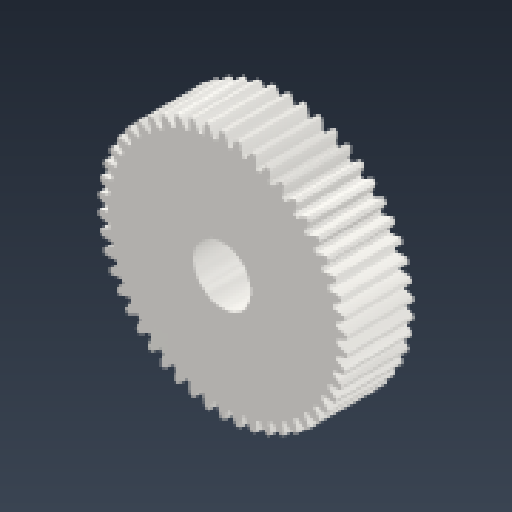
# Autodesk Inventor part: Цилиндрическое зубчатое зацепление1
Saved by Autodesk Inventor 2025 (Build 290162000, 162)
## iProperties
Created: 2025-09-21
Part Number: Цилиндрическое зубчатое зацепление1
Material: Steel
Document SubType Name: Modeling
Designer: GameHD
Categories: <?xml version="1.0" encoding="UTF-16"?> <MemberInstance><Categories><FamilyTemplate><FamilyTemplateParameter ValueType="xs:double" Id="1" ObjectReferenceKey="da_z" ObjectType="kUserParameterObject"/><FamilyTemplateParameter ValueType="xs:double" Id="2" ObjectReferenceKey="da_b" ObjectType="kUserParameterObject"/><FamilyTemplateParameter ValueType="xs:double" Id="3" ObjectReferenceKey="da_beta" ObjectType="kUserParameterObject"/><FamilyTemplateParameter ValueType="xs:double" Id="4" ObjectReferenceKey="da_da" ObjectType="kUserParameterObject"/><FamilyTemplateParameter ValueType="xs:double" Id="5" ObjectReferenceKey="da_aw" ObjectType="kUserParameterObject"/><FamilyTemplateParameter ValueType="xs:string" Id="6" ObjectReferenceKey="EAIAABAAAACIAQAAAAAAAIAAAAAAAAAA" ObjectType="83910656" SubObjectId="SurfaceGeometry"/></FamilyTemplate><ParamToTemplateMap><ParamToTemplate CategoryParameter="//CategoryParameter[@InternalName='046C89C9-8512-4d59-83FE-43B91F4F132A']" TemplateParameter="1"/><ParamToTemplate CategoryParameter="//CategoryParameter[@InternalName='2552DF32-E462-4b46-AEBF-C6C7768E72AC']" TemplateParameter="2"/><ParamToTemplate CategoryParameter="//CategoryParameter[@InternalName='C9EE641D-15FC-4fae-A226-E94C4372FDD7']" TemplateParameter="3"/><ParamToTemplate><ParamToTemplate CategoryParameter="//CategoryParameter[@InternalName='00B6519A-459B-49c7-AD84-2E56D39A5744']" ConstantValue="0.000000"/></ParamToTemplate><ParamToTemplate><ParamToTemplate CategoryParameter="//CategoryParameter[@InternalName='04B31F0E-C7A6-4894-AA32-9629BEFACF47']" ConstantValue="1.000000"/></ParamToTemplate><ParamToTemplate><ParamToTemplate CategoryParameter="//CategoryParameter[@InternalName='43CBEC2E-7847-49e7-A936-2F7889FCB2D9']" ConstantValue="0.250000"/></ParamToTemplate><ParamToTemplate><ParamToTemplate CategoryParameter="//CategoryParameter[@InternalName='B1EFC894-105D-4ebd-86BF-FA20ED196853']" ConstantValue="0.350000"/></ParamToTemplate><ParamToTemplate><ParamToTemplate CategoryParameter="//CategoryParameter[@InternalName='51175063-3D10-4879-93E8-6246FE8B403D']" ConstantValue="2060000000.000000"/></ParamToTemplate><ParamToTemplate><ParamToTemplate CategoryParameter="//CategoryParameter[@InternalName='A3A52E27-4454-46a9-B0BD-C932399B70AF']" ConstantValue="0.300000"/></ParamToTemplate><ParamToTemplate><ParamToTemplate CategoryParameter="//CategoryParameter[@InternalName='91B76062-C214-41d9-B1B9-14D2AB99603D']" ConstantValue="0.050000"/></ParamToTemplate><ParamToTemplate><ParamToTemplate CategoryParameter="//CategoryParameter[@InternalName='374E806E-8B8A-4dda-A9AA-1039D6500AD2']" ConstantValue="20.000000"/></ParamToTemplate><ParamToTemplate><ParamToTemplate CategoryParameter="//CategoryParameter[@InternalName='2D373A89-B862-43d6-8D0B-0CBF12AB9F6C']" ConstantValue="0.349066"/></ParamToTemplate><ParamToTemplate CategoryParameter="//CategoryParameter[@InternalName='37777632-D6A2-4fac-9D53-DB8ACD95C989']" TemplateParameter="4"/><ParamToTemplate CategoryParameter="//CategoryParameter[@InternalName='FD1017F1-B727-4f7e-9707-0F86F1FF9423']" TemplateParameter="5"/><ParamToTemplate><ParamToTemplate CategoryParameter="//CategoryParameter[@InternalName='9E1B4470-B2D3-4ff1-B813-535BB4CDF51A']" ConstantValue="3520000.000000"/></ParamToTemplate><ParamToTemplate><ParamToTemplate CategoryParameter="//CategoryParameter[@InternalName='F8452263-BFF6-458c-9FB1-07C4B99E95CD']" ConstantValue="11400000.000000"/></ParamToTemplate><ParamToTemplate><ParamToTemplate CategoryParameter="//CategoryParameter[@InternalName='3E3BB259-FD49-497f-8171-6EBC954A3479']" ConstantValue="2.000000"/></ParamToTemplate><ParamToTemplate CategoryParameter="//CategoryParameter[@InternalName='27C3BAF2-7550-4e4b-AE2C-0DB134B7D9B7']" TemplateParameter="6"/></ParamToTemplateMap><Category DisplayName="Gear" InternalName="DC85795E-93AB-48d5-8EEE-5A27447B64BD" Mnemonic="Gear"><CategoryParameter DisplayName="z" InternalName="046C89C9-8512-4d59-83FE-43B91F4F132A" Mnemonic="z"/><CategoryParameter DisplayName="b" InternalName="2552DF32-E462-4b46-AEBF-C6C7768E72AC" Mnemonic="b"/><CategoryParameter DisplayName="||b|" InternalName="C9EE641D-15FC-4fae-A226-E94C4372FDD7" Mnemonic="beta"/><CategoryParameter DisplayName="x" InternalName="00B6519A-459B-49c7-AD84-2E56D39A5744" Mnemonic="x"/><CategoryParameter DisplayName="a*" InternalName="04B31F0E-C7A6-4894-AA32-9629BEFACF47" Mnemonic="a"/><CategoryParameter DisplayName="c*" InternalName="43CBEC2E-7847-49e7-A936-2F7889FCB2D9" Mnemonic="c"/><CategoryParameter DisplayName="r|.f|*" InternalName="B1EFC894-105D-4ebd-86BF-FA20ED196853" Mnemonic="rf"/><CategoryParameter DisplayName="E" InternalName="51175063-3D10-4879-93E8-6246FE8B403D" Mnemonic="E"/><CategoryParameter DisplayName="||m|" InternalName="A3A52E27-4454-46a9-B0BD-C932399B70AF" Mnemonic="mi"/><Category DisplayName="SpurGear" InternalName="26C5A22E-A91E-4dfd-A3B3-23CCAFAE1764" Mnemonic="SpurGear"><CategoryParameter DisplayName="m" InternalName="91B76062-C214-41d9-B1B9-14D2AB99603D" Mnemonic="m"/><CategoryParameter DisplayName="P" InternalName="374E806E-8B8A-4dda-A9AA-1039D6500AD2" Mnemonic="PP"/><CategoryParameter DisplayName="||a|" InternalName="2D373A89-B862-43d6-8D0B-0CBF12AB9F6C" Mnemonic="alpha"/><CategoryParameter DisplayName="d|.a|" InternalName="37777632-D6A2-4fac-9D53-DB8ACD95C989" Mnemonic="da"/><CategoryParameter DisplayName="a|.w|" InternalName="FD1017F1-B727-4f7e-9707-0F86F1FF9423" Mnemonic="aw"/><CategoryParameter DisplayName="||s||.Flim|" InternalName="9E1B4470-B2D3-4ff1-B813-535BB4CDF51A" Mnemonic="sFlim"/><CategoryParameter DisplayName="||s||.Hlim|" InternalName="F8452263-BFF6-458c-9FB1-07C4B99E95CD" Mnemonic="sHlim"/><CategoryParameter DisplayName="тип" InternalName="3E3BB259-FD49-497f-8171-6EBC954A3479" Mnemonic="type"/><CategoryParameter DisplayName="PitchDiameter" InternalName="27C3BAF2-7550-4e4b-AE2C-0DB134B7D9B7" Mnemonic="IDS_PITCHDIAM"/></Category></Category></Categories></MemberInstance>
Density: 1 g/cm^3
Appearance: Steel
CustomPartVersion: 1
Author: GameHD
Autodesk Inventor part; units mm, degrees
sketch "Sketch1" plane through (0, 0, 0) normal (0, 0, 1) x (1, 0, 0)
  circle A0 centre (0, 0) radius 13
  dimension "d0" = 26
  constraints: 1 centre point
  measures "d0" diameter of A0
extrude "Extrusion1" add sketch "Sketch1" along normal blind 6.5
ref_plane "Work Plane2" through (0, 0, 3.25) normal (0, 0, 1) x (1, 0, 0)
sketch "Sketch2" plane through (0, 0, 0) normal (0, 0, -1) x (-1, 0, 0)
  circle A0 centre (0, 0) radius 13 projected
  circle A1 centre (0, 0) radius 12.5
  dimension "d3" = 25
  constraints: 1 centre point, 1 coincident
  measures "d3" diameter of A1
surface extrude "Средний диаметр" sketch "Sketch2" against normal through all shown no curves A1
ref_plane "Work Plane8" through (0, 0, 0) normal (0.9980267, 0.0627905, 0) x (0, 0, 1)
ref_plane "Work Plane9" through (0, 0, 0) normal (1, 0, 0) x (0, 1, 0)
spur gear teeth "Цилиндрическое зубчатое зацепление" teeth 50 pitch diameter 25 tip diameter 26 root diameter 23.75 face width 6.5 start plane through (0, 0, 0) normal (0, 0, -1) x (-1, 0, 0)
sketch "Эскиз3" plane through (0, 0, 6.5) normal (0, 0, 1) x (1, 0, 0)
  circle A0 centre (0, 0) radius 3
  dimension "d49" = 6
  constraints: 1 centre point, 1 coincident
  measures "d49" diameter of A0
extrude "Выдавливание2" cut sketch "Эскиз3" against normal blind 10
sketch "Эскиз4" plane through (0, 0, 6.5) normal (0, 0, 1) x (1, 0, 0)
  circle A0 centre (0, 0) radius 4.5
  circle A1 centre (0, 0) radius 3 projected
  dimension "d52" = 9
  constraints: 1 centre point, 1 coincident
  measures "d52" diameter of A0
extrude "Выдавливание3" add sketch "Эскиз4" along normal blind 1
sketch "Эскиз5" plane through (0, 0, 0) normal (0, 0, -1) x (-1, 0, 0)
  circle A0 centre (0, 0) radius 4.5 projected
  circle A1 centre (0, 0) radius 3 projected
  arc A2 (2.0417, 11.6982) -> (1.8317, 12.8703) centre (-3.9363, 11.2323) ccw projected
  arc A3 (1.8317, 12.8703) -> (1.4265, 12.9215) centre (0, 0) ccw projected
  arc A4 (1.4265, 12.9215) -> (0.9317, 11.8384) centre (6.606, 9.9005) ccw projected
  arc A5 (0.9317, 11.8384) -> (0.5594, 11.8618) centre (0, 0) ccw projected
  arc A6 (0.5594, 11.8618) -> (0.2042, 12.9984) centre (-5.313, 10.6504) ccw projected
  arc A7 (0.2042, 12.9984) -> (-0.2042, 12.9984) centre (0, 0) ccw projected
  arc A8 (-0.2042, 12.9984) -> (-0.5594, 11.8618) centre (5.313, 10.6504) ccw projected
  arc A9 (-0.5594, 11.8618) -> (-0.9317, 11.8384) centre (0, 0) ccw projected
  arc A10 (-0.9317, 11.8384) -> (-1.4265, 12.9215) centre (-6.606, 9.9005) ccw projected
  arc A11 (-1.4265, 12.9215) -> (-1.8317, 12.8703) centre (0, 0) ccw projected
  arc A12 (-1.8317, 12.8703) -> (-2.0417, 11.6982) centre (3.9363, 11.2323) ccw projected
  arc A13 (-2.0417, 11.6982) -> (-2.4081, 11.6283) centre (0, 0) ccw projected
  arc A14 (-2.4081, 11.6283) -> (-3.0348, 12.6408) centre (-7.7948, 8.9945) ccw projected
  arc A15 (-3.0348, 12.6408) -> (-3.4303, 12.5392) centre (0, 0) ccw projected
  arc A16 (-3.4303, 12.5392) -> (-3.4917, 11.35) centre (2.4975, 11.6371) ccw projected
  arc A17 (-3.4917, 11.35) -> (-3.8465, 11.2348) centre (0, 0) ccw projected
  arc A18 (-3.8465, 11.2348) -> (-4.5952, 12.1608) centre (-8.8606, 7.9466) ccw projected
  arc A19 (-4.5952, 12.1608) -> (-4.9749, 12.0104) centre (0, 0) ccw projected
  arc A20 (-4.9749, 12.0104) -> (-4.8867, 10.8229) centre (1.0193, 11.8584) ccw projected
  arc A21 (-4.8867, 10.8229) -> (-5.2243, 10.6641) centre (0, 0) ccw projected
  arc A22 (-5.2243, 10.6641) -> (-6.0831, 11.489) centre (-9.7867, 6.7734) ccw projected
  arc A23 (-6.0831, 11.489) -> (-6.441, 11.2922) centre (0, 0) ccw projected
  arc A24 (-6.441, 11.2922) -> (-6.2047, 10.1251) centre (-0.475, 11.8926) ccw projected
  arc A25 (-6.2047, 10.1251) -> (-6.5196, 9.9252) centre (0, 0) ccw projected
  arc A26 (-6.5196, 9.9252) -> (-7.4751, 10.6359) centre (-10.5585, 5.4934) ccw projected
  arc A27 (-7.4751, 10.6359) -> (-7.8055, 10.3959) centre (0, 0) ccw projected
  arc A28 (-7.8055, 10.3959) -> (-7.4248, 9.2676) centre (-1.9618, 11.7393) ccw projected
  arc A29 (-7.4248, 9.2676) -> (-7.7122, 9.0298) centre (0, 0) ccw projected
  arc A30 (-7.7122, 9.0298) -> (-8.7492, 9.6152) centre (-11.1637, 4.1268) ccw projected
  arc A31 (-8.7492, 9.6152) -> (-9.0469, 9.3356) centre (0, 0) ccw projected
  arc A32 (-9.0469, 9.3356) -> (-8.5277, 8.264) centre (-3.4177, 11.4008) ccw projected
  arc A33 (-8.5277, 8.264) -> (-8.7831, 7.992) centre (0, 0) ccw projected
  arc A34 (-8.7831, 7.992) -> (-9.8853, 8.4428) centre (-11.5929, 2.6951) ccw projected
  arc A35 (-9.8853, 8.4428) -> (-10.1456, 8.1282) centre (0, 0) ccw projected
  arc A36 (-10.1456, 8.1282) -> (-9.4963, 7.13) centre (-4.8196, 10.8826) ccw projected
  arc A37 (-9.4963, 7.13) -> (-9.7155, 6.8282) centre (0, 0) ccw projected
  arc A38 (-9.7155, 6.8282) -> (-10.8655, 7.1373) centre (-11.8393, 1.2208) ccw projected
  arc A39 (-10.8655, 7.1373) -> (-11.0843, 6.7925) centre (0, 0) ccw projected
  arc A40 (-11.0843, 6.7925) -> (-10.315, 5.8836) centre (-6.1456, 10.1927) ccw projected
  arc A41 (-10.315, 5.8836) -> (-10.4947, 5.5567) centre (0, 0) ccw projected
  arc A42 (-10.4947, 5.5567) -> (-11.6744, 5.7192) centre (-11.899, -0.2727) ccw projected
  arc A43 (-11.6744, 5.7192) -> (-11.8482, 5.3497) centre (0, 0) ccw projected
  arc A44 (-11.8482, 5.3497) -> (-10.9711, 4.5444) centre (-7.3746, 9.3421) ccw projected
  arc A45 (-10.9711, 4.5444) -> (-11.1084, 4.1975) centre (0, 0) ccw projected
  arc A46 (-11.1084, 4.1975) -> (-12.2991, 4.2109) centre (-11.771, -1.7619) ccw projected
  arc A47 (-12.2991, 4.2109) -> (-12.4253, 3.8225) centre (0, 0) ccw projected
  arc A48 (-12.4253, 3.8225) -> (-11.4541, 3.1335) centre (-8.4873, 8.3442) ccw projected
  arc A49 (-11.4541, 3.1335) -> (-11.5469, 2.7722) centre (0, 0) ccw projected
  arc A50 (-11.5469, 2.7722) -> (-12.7299, 2.6362) centre (-11.4573, -3.2233) ccw projected
  arc A51 (-12.7299, 2.6362) -> (-12.8064, 2.2351) centre (0, 0) ccw projected
  arc A52 (-12.8064, 2.2351) -> (-11.7565, 1.6732) centre (-9.4662, 7.2146) ccw projected
  arc A53 (-11.7565, 1.6732) -> (-11.8033, 1.3031) centre (0, 0) ccw projected
  arc A54 (-11.8033, 1.3031) -> (-12.9599, 1.02) centre (-10.963, -4.6338) ccw projected
  arc A55 (-12.9599, 1.02) -> (-12.9856, 0.6124) centre (0, 0) ccw projected
  arc A56 (-12.9856, 0.6124) -> (-11.8735, 0.1865) centre (-10.2958, 5.9713) ccw projected
  arc A57 (-11.8735, 0.1865) -> (-11.8735, -0.1865) centre (0, 0) ccw projected
  arc A58 (-11.8735, -0.1865) -> (-12.9856, -0.6124) centre (-10.2958, -5.9713) ccw projected
  arc A59 (-12.9856, -0.6124) -> (-12.9599, -1.02) centre (0, 0) ccw projected
  arc A60 (-12.9599, -1.02) -> (-11.8033, -1.3031) centre (-10.963, 4.6338) ccw projected
  arc A61 (-11.8033, -1.3031) -> (-11.7565, -1.6732) centre (0, 0) ccw projected
  arc A62 (-11.7565, -1.6732) -> (-12.8064, -2.2351) centre (-9.4662, -7.2146) ccw projected
  arc A63 (-12.8064, -2.2351) -> (-12.7299, -2.6362) centre (0, 0) ccw projected
  arc A64 (-12.7299, -2.6362) -> (-11.5469, -2.7722) centre (-11.4573, 3.2233) ccw projected
  arc A65 (-11.5469, -2.7722) -> (-11.4541, -3.1335) centre (0, 0) ccw projected
  arc A66 (-11.4541, -3.1335) -> (-12.4253, -3.8225) centre (-8.4873, -8.3442) ccw projected
  arc A67 (-12.4253, -3.8225) -> (-12.2991, -4.2109) centre (0, 0) ccw projected
  arc A68 (-12.2991, -4.2109) -> (-11.1084, -4.1975) centre (-11.771, 1.7619) ccw projected
  arc A69 (-11.1084, -4.1975) -> (-10.9711, -4.5444) centre (0, 0) ccw projected
  arc A70 (-10.9711, -4.5444) -> (-11.8482, -5.3497) centre (-7.3746, -9.3421) ccw projected
  arc A71 (-11.8482, -5.3497) -> (-11.6744, -5.7192) centre (0, 0) ccw projected
  arc A72 (-11.6744, -5.7192) -> (-10.4947, -5.5567) centre (-11.899, 0.2727) ccw projected
  arc A73 (-10.4947, -5.5567) -> (-10.315, -5.8836) centre (0, 0) ccw projected
  arc A74 (-10.315, -5.8836) -> (-11.0843, -6.7925) centre (-6.1456, -10.1927) ccw projected
  arc A75 (-11.0843, -6.7925) -> (-10.8655, -7.1373) centre (0, 0) ccw projected
  arc A76 (-10.8655, -7.1373) -> (-9.7155, -6.8282) centre (-11.8393, -1.2208) ccw projected
  arc A77 (-9.7155, -6.8282) -> (-9.4963, -7.13) centre (0, 0) ccw projected
  arc A78 (-9.4963, -7.13) -> (-10.1456, -8.1282) centre (-4.8196, -10.8826) ccw projected
  arc A79 (-10.1456, -8.1282) -> (-9.8853, -8.4428) centre (0, 0) ccw projected
  arc A80 (-9.8853, -8.4428) -> (-8.7831, -7.992) centre (-11.5929, -2.6951) ccw projected
  arc A81 (-8.7831, -7.992) -> (-8.5277, -8.264) centre (0, 0) ccw projected
  arc A82 (-8.5277, -8.264) -> (-9.0469, -9.3356) centre (-3.4177, -11.4008) ccw projected
  arc A83 (-9.0469, -9.3356) -> (-8.7492, -9.6152) centre (0, 0) ccw projected
  arc A84 (-8.7492, -9.6152) -> (-7.7122, -9.0298) centre (-11.1637, -4.1268) ccw projected
  arc A85 (-7.7122, -9.0298) -> (-7.4248, -9.2676) centre (0, 0) ccw projected
  arc A86 (-7.4248, -9.2676) -> (-7.8055, -10.3959) centre (-1.9618, -11.7393) ccw projected
  arc A87 (-7.8055, -10.3959) -> (-7.4751, -10.6359) centre (0, 0) ccw projected
  arc A88 (-7.4751, -10.6359) -> (-6.5196, -9.9252) centre (-10.5585, -5.4934) ccw projected
  arc A89 (-6.5196, -9.9252) -> (-6.2047, -10.1251) centre (0, 0) ccw projected
  arc A90 (-6.2047, -10.1251) -> (-6.441, -11.2922) centre (-0.475, -11.8926) ccw projected
  arc A91 (-6.441, -11.2922) -> (-6.0831, -11.489) centre (0, 0) ccw projected
  arc A92 (-6.0831, -11.489) -> (-5.2243, -10.6641) centre (-9.7867, -6.7734) ccw projected
  arc A93 (-5.2243, -10.6641) -> (-4.8867, -10.8229) centre (0, 0) ccw projected
  arc A94 (-4.8867, -10.8229) -> (-4.9749, -12.0104) centre (1.0193, -11.8584) ccw projected
  arc A95 (-4.9749, -12.0104) -> (-4.5952, -12.1608) centre (0, 0) ccw projected
  arc A96 (-4.5952, -12.1608) -> (-3.8465, -11.2348) centre (-8.8606, -7.9466) ccw projected
  arc A97 (-3.8465, -11.2348) -> (-3.4917, -11.35) centre (0, 0) ccw projected
  arc A98 (-3.4917, -11.35) -> (-3.4303, -12.5392) centre (2.4975, -11.6371) ccw projected
  arc A99 (-3.4303, -12.5392) -> (-3.0348, -12.6408) centre (0, 0) ccw projected
  arc A100 (-3.0348, -12.6408) -> (-2.4081, -11.6283) centre (-7.7948, -8.9945) ccw projected
  arc A101 (-2.4081, -11.6283) -> (-2.0417, -11.6982) centre (0, 0) ccw projected
  arc A102 (-2.0417, -11.6982) -> (-1.8317, -12.8703) centre (3.9363, -11.2323) ccw projected
  arc A103 (-1.8317, -12.8703) -> (-1.4265, -12.9215) centre (0, 0) ccw projected
  arc A104 (-1.4265, -12.9215) -> (-0.9317, -11.8384) centre (-6.606, -9.9005) ccw projected
  arc A105 (-0.9317, -11.8384) -> (-0.5594, -11.8618) centre (0, 0) ccw projected
  arc A106 (-0.5594, -11.8618) -> (-0.2042, -12.9984) centre (5.313, -10.6504) ccw projected
  arc A107 (-0.2042, -12.9984) -> (0.2042, -12.9984) centre (0, 0) ccw projected
  arc A108 (0.2042, -12.9984) -> (0.5594, -11.8618) centre (-5.313, -10.6504) ccw projected
  arc A109 (0.5594, -11.8618) -> (0.9317, -11.8384) centre (0, 0) ccw projected
  arc A110 (0.9317, -11.8384) -> (1.4265, -12.9215) centre (6.606, -9.9005) ccw projected
  arc A111 (1.4265, -12.9215) -> (1.8317, -12.8703) centre (0, 0) ccw projected
  arc A112 (1.8317, -12.8703) -> (2.0417, -11.6982) centre (-3.9363, -11.2323) ccw projected
  arc A113 (2.0417, -11.6982) -> (2.4081, -11.6283) centre (0, 0) ccw projected
  arc A114 (2.4081, -11.6283) -> (3.0348, -12.6408) centre (7.7948, -8.9945) ccw projected
  arc A115 (3.0348, -12.6408) -> (3.4303, -12.5392) centre (0, 0) ccw projected
  arc A116 (3.4303, -12.5392) -> (3.4917, -11.35) centre (-2.4975, -11.6371) ccw projected
  arc A117 (3.4917, -11.35) -> (3.8465, -11.2348) centre (0, 0) ccw projected
  arc A118 (3.8465, -11.2348) -> (4.5952, -12.1608) centre (8.8606, -7.9466) ccw projected
  arc A119 (4.5952, -12.1608) -> (4.9749, -12.0104) centre (0, 0) ccw projected
  arc A120 (4.9749, -12.0104) -> (4.8867, -10.8229) centre (-1.0193, -11.8584) ccw projected
  arc A121 (4.8867, -10.8229) -> (5.2243, -10.6641) centre (0, 0) ccw projected
  arc A122 (5.2243, -10.6641) -> (6.0831, -11.489) centre (9.7867, -6.7734) ccw projected
  arc A123 (6.0831, -11.489) -> (6.441, -11.2922) centre (0, 0) ccw projected
  arc A124 (6.441, -11.2922) -> (6.2047, -10.1251) centre (0.475, -11.8926) ccw projected
  arc A125 (6.2047, -10.1251) -> (6.5196, -9.9252) centre (0, 0) ccw projected
  arc A126 (6.5196, -9.9252) -> (7.4751, -10.6359) centre (10.5585, -5.4934) ccw projected
  arc A127 (7.4751, -10.6359) -> (7.8055, -10.3959) centre (0, 0) ccw projected
  arc A128 (7.8055, -10.3959) -> (7.4248, -9.2676) centre (1.9618, -11.7393) ccw projected
  arc A129 (7.4248, -9.2676) -> (7.7122, -9.0298) centre (0, 0) ccw projected
  arc A130 (7.7122, -9.0298) -> (8.7492, -9.6152) centre (11.1637, -4.1268) ccw projected
  arc A131 (8.7492, -9.6152) -> (9.0469, -9.3356) centre (0, 0) ccw projected
  arc A132 (9.0469, -9.3356) -> (8.5277, -8.264) centre (3.4177, -11.4008) ccw projected
  arc A133 (8.5277, -8.264) -> (8.7831, -7.992) centre (0, 0) ccw projected
  arc A134 (8.7831, -7.992) -> (9.8853, -8.4428) centre (11.5929, -2.6951) ccw projected
  arc A135 (9.8853, -8.4428) -> (10.1456, -8.1282) centre (0, 0) ccw projected
  arc A136 (10.1456, -8.1282) -> (9.4963, -7.13) centre (4.8196, -10.8826) ccw projected
  arc A137 (9.4963, -7.13) -> (9.7155, -6.8282) centre (0, 0) ccw projected
  arc A138 (9.7155, -6.8282) -> (10.8655, -7.1373) centre (11.8393, -1.2208) ccw projected
  arc A139 (10.8655, -7.1373) -> (11.0843, -6.7925) centre (0, 0) ccw projected
  arc A140 (11.0843, -6.7925) -> (10.315, -5.8836) centre (6.1456, -10.1927) ccw projected
  arc A141 (10.315, -5.8836) -> (10.4947, -5.5567) centre (0, 0) ccw projected
  arc A142 (10.4947, -5.5567) -> (11.6744, -5.7192) centre (11.899, 0.2727) ccw projected
  arc A143 (11.6744, -5.7192) -> (11.8482, -5.3497) centre (0, 0) ccw projected
  arc A144 (11.8482, -5.3497) -> (10.9711, -4.5444) centre (7.3746, -9.3421) ccw projected
  arc A145 (10.9711, -4.5444) -> (11.1084, -4.1975) centre (0, 0) ccw projected
  arc A146 (11.1084, -4.1975) -> (12.2991, -4.2109) centre (11.771, 1.7619) ccw projected
  arc A147 (12.2991, -4.2109) -> (12.4253, -3.8225) centre (0, 0) ccw projected
  arc A148 (12.4253, -3.8225) -> (11.4541, -3.1335) centre (8.4873, -8.3442) ccw projected
  arc A149 (11.4541, -3.1335) -> (11.5469, -2.7722) centre (0, 0) ccw projected
  arc A150 (11.5469, -2.7722) -> (12.7299, -2.6362) centre (11.4573, 3.2233) ccw projected
  arc A151 (12.7299, -2.6362) -> (12.8064, -2.2351) centre (0, 0) ccw projected
  arc A152 (12.8064, -2.2351) -> (11.7565, -1.6732) centre (9.4662, -7.2146) ccw projected
  arc A153 (11.7565, -1.6732) -> (11.8033, -1.3031) centre (0, 0) ccw projected
  arc A154 (11.8033, -1.3031) -> (12.9599, -1.02) centre (10.963, 4.6338) ccw projected
  arc A155 (12.9599, -1.02) -> (12.9856, -0.6124) centre (0, 0) ccw projected
  arc A156 (12.9856, -0.6124) -> (11.8735, -0.1865) centre (10.2958, -5.9713) ccw projected
  arc A157 (11.8735, -0.1865) -> (11.8735, 0.1865) centre (0, 0) ccw projected
  arc A158 (11.8735, 0.1865) -> (12.9856, 0.6124) centre (10.2958, 5.9713) ccw projected
  arc A159 (12.9856, 0.6124) -> (12.9599, 1.02) centre (0, 0) ccw projected
  arc A160 (12.9599, 1.02) -> (11.8033, 1.3031) centre (10.963, -4.6338) ccw projected
  arc A161 (11.8033, 1.3031) -> (11.7565, 1.6732) centre (0, 0) ccw projected
  arc A162 (11.7565, 1.6732) -> (12.8064, 2.2351) centre (9.4662, 7.2146) ccw projected
  arc A163 (12.8064, 2.2351) -> (12.7299, 2.6362) centre (0, 0) ccw projected
  arc A164 (12.7299, 2.6362) -> (11.5469, 2.7722) centre (11.4573, -3.2233) ccw projected
  arc A165 (11.5469, 2.7722) -> (11.4541, 3.1335) centre (0, 0) ccw projected
  arc A166 (11.4541, 3.1335) -> (12.4253, 3.8225) centre (8.4873, 8.3442) ccw projected
  arc A167 (12.4253, 3.8225) -> (12.2991, 4.2109) centre (0, 0) ccw projected
  arc A168 (12.2991, 4.2109) -> (11.1084, 4.1975) centre (11.771, -1.7619) ccw projected
  arc A169 (11.1084, 4.1975) -> (10.9711, 4.5444) centre (0, 0) ccw projected
  arc A170 (10.9711, 4.5444) -> (11.8482, 5.3497) centre (7.3746, 9.3421) ccw projected
  arc A171 (11.8482, 5.3497) -> (11.6744, 5.7192) centre (0, 0) ccw projected
  arc A172 (11.6744, 5.7192) -> (10.4947, 5.5567) centre (11.899, -0.2727) ccw projected
  arc A173 (10.4947, 5.5567) -> (10.315, 5.8836) centre (0, 0) ccw projected
  arc A174 (10.315, 5.8836) -> (11.0843, 6.7925) centre (6.1456, 10.1927) ccw projected
  arc A175 (11.0843, 6.7925) -> (10.8655, 7.1373) centre (0, 0) ccw projected
  arc A176 (10.8655, 7.1373) -> (9.7155, 6.8282) centre (11.8393, 1.2208) ccw projected
  arc A177 (9.7155, 6.8282) -> (9.4963, 7.13) centre (0, 0) ccw projected
  arc A178 (9.4963, 7.13) -> (10.1456, 8.1282) centre (4.8196, 10.8826) ccw projected
  arc A179 (10.1456, 8.1282) -> (9.8853, 8.4428) centre (0, 0) ccw projected
  arc A180 (9.8853, 8.4428) -> (8.7831, 7.992) centre (11.5929, 2.6951) ccw projected
  arc A181 (8.7831, 7.992) -> (8.5277, 8.264) centre (0, 0) ccw projected
  arc A182 (8.5277, 8.264) -> (9.0469, 9.3356) centre (3.4177, 11.4008) ccw projected
  arc A183 (9.0469, 9.3356) -> (8.7492, 9.6152) centre (0, 0) ccw projected
  arc A184 (8.7492, 9.6152) -> (7.7122, 9.0298) centre (11.1637, 4.1268) ccw projected
  arc A185 (7.7122, 9.0298) -> (7.4248, 9.2676) centre (0, 0) ccw projected
  arc A186 (7.4248, 9.2676) -> (7.8055, 10.3959) centre (1.9618, 11.7393) ccw projected
  arc A187 (7.8055, 10.3959) -> (7.4751, 10.6359) centre (0, 0) ccw projected
  arc A188 (7.4751, 10.6359) -> (6.5196, 9.9252) centre (10.5585, 5.4934) ccw projected
  arc A189 (6.5196, 9.9252) -> (6.2047, 10.1251) centre (0, 0) ccw projected
  arc A190 (6.2047, 10.1251) -> (6.441, 11.2922) centre (0.475, 11.8926) ccw projected
  arc A191 (6.441, 11.2922) -> (6.0831, 11.489) centre (0, 0) ccw projected
  arc A192 (6.0831, 11.489) -> (5.2243, 10.6641) centre (9.7867, 6.7734) ccw projected
  arc A193 (5.2243, 10.6641) -> (4.8867, 10.8229) centre (0, 0) ccw projected
  arc A194 (4.8867, 10.8229) -> (4.9749, 12.0104) centre (-1.0193, 11.8584) ccw projected
  arc A195 (4.9749, 12.0104) -> (4.5952, 12.1608) centre (0, 0) ccw projected
  arc A196 (4.5952, 12.1608) -> (3.8465, 11.2348) centre (8.8606, 7.9466) ccw projected
  arc A197 (3.8465, 11.2348) -> (3.4917, 11.35) centre (0, 0) ccw projected
  arc A198 (3.4917, 11.35) -> (3.4303, 12.5392) centre (-2.4975, 11.6371) ccw projected
  arc A199 (3.4303, 12.5392) -> (3.0348, 12.6408) centre (0, 0) ccw projected
  arc A200 (3.0348, 12.6408) -> (2.4081, 11.6283) centre (7.7948, 8.9945) ccw projected
  arc A201 (2.4081, 11.6283) -> (2.0417, 11.6982) centre (0, 0) ccw projected
extrude "Выдавливание4" add sketch "Эскиз5" along normal blind 1 contours A0
equation "\"d0\" = da_da"
equation "\"d1\" = da_b"
equation "\"d3\" = da_d"
equation "\"d16\" = da_aw"
equation "\"d43\" = da_aw"
equation "\"d46\" = da_aw"
equation "\"da_da\" = 26"
equation "\"da_b\" = 6.5"
equation "\"da_d\" = 25"
equation "\"da_aw\" = 43.5"
body "Solid1"
body "Srf1"
